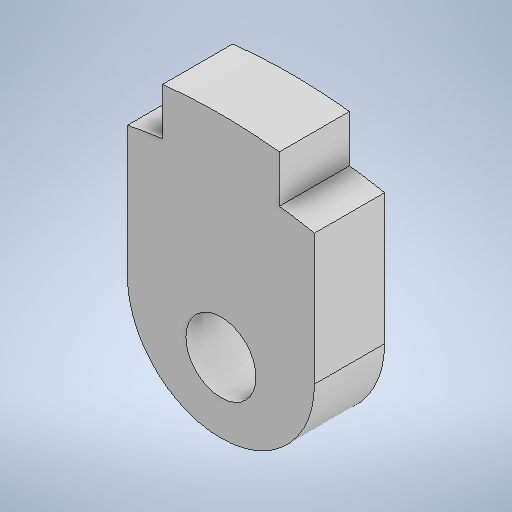
# Autodesk Inventor part: ModuleConnector_Outside_Axis
Saved by Autodesk Inventor 2025.1 (Build 291241020, 241B)
## iProperties
Created: 2024-10-09
Part Number: ModuleConnector_Outside_Axis
Material: 일반
Document SubType Name: Modeling
Designer: SEON06
Density: 1 g/cm^3
Appearance: 기본값
Author: SEON06
Autodesk Inventor part; units mm, degrees
ref_plane "YZ Plane" through (0, 0, 0) normal (1, 0, 0) x (0, 1, 0)
ref_plane "XZ Plane" through (0, 0, 0) normal (0, 1, 0) x (-1, 0, 0)
ref_plane "XY Plane" through (0, 0, 0) normal (0, 0, 1) x (1, 0, 0)
sketch "스케치1" plane through (0, 0, 0) normal (0, 0, 1) x (1, 0, 0)
  circle A0 centre (0, 0) radius 20
  line L0 (-4, 19.5959) -> (-4, 0)
  line L1 (-4, 0) -> (4, 0)
  line L2 (4, 0) -> (4, 19.5959)
  circle A1 centre (0, 0) radius 10
  line L3 (-2.5, 21.8575) -> (-2.5, 19.8431)
  line L4 (2.5, 21.8575) -> (2.5, 19.8431)
  circle A2 centre (0, 0) radius 22
  point P0 (0, 0)
  point P1 (0, 0)
  point P2 (-4, 9.1652)
  point P3 (4, 9.1652)
  dimension "d0" = 40
  dimension "d1" = 8
  dimension "d5" = 20
  dimension "d13" = 2
  dimension "d14" = 5
  dimension "d15" = 2.5
  constraints: 10 end point, 6 point on circle, 5 coincident, 3 centre point, 3 vertical, 2 perpendicular, 1 midpoint
  measures "d0" diameter of A0
  measures "d1" distance of L0.end L1.end
  measures "d5" diameter of A1
  measures "d13" radial gap between concentric circles of A0 A2
  measures "d14" distance between parallel lines of L4 L3
  measures "d15" distance from line of point (0, 0) L3
extrude "돌출1" add sketch "스케치1" along normal blind 3 contours L2 A1 L0 A0 | A0 L3 A2 L4 picked at (-1.5144, 13.2107) picked at (-1.9451, 20.5611)
sketch "스케치2" plane through (0, 0, 3) normal (0, 0, 1) x (1, 0, 0)
  circle A0 centre (0, 13) radius 1.5
  arc A1 (4, 9.1652) -> (-4, 9.1652) centre (0, 0) ccw projected
  point P0 (0, 0)
  point P1 (0, 10)
  dimension "d6" = 3
  dimension "d7" = 3
  constraints: 1 centre point, 1 point on circle, 1 vertical alignment
  measures "d6" diameter of A0
  measures "d7" distance of point (0, 10) A0.centre
extrude "돌출2" cut sketch "스케치2" against normal through all
fillet "모깎기1" radius 4 2 edges at (-4, 9.1652, 1.5) (4, 9.1652, 1.5)
equation "\"d15\" = 0.5 * d14"
